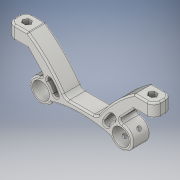
# Autodesk Inventor part: Carbon fibre tube front bracket 3.0
Saved by Autodesk Inventor 2016 (Build 200138000, 138)
## iProperties
Created: 2016-01-16
Part Number: Carbon fibre tube front bracket 3.0
Material: Generic
Document SubType Name: Modeling
Designer: Josiah Stark
Density: 1 g/cm^3
Appearance: Default
Author: Josiah Stark
Autodesk Inventor part; units mm, degrees
ref_plane "YZ Plane" through (0, 0, 0) normal (1, 0, 0) x (0, 1, 0)
sketch "Sketch1" plane through (0, 0, 0) normal (0, 0, 1) x (1, 0, 0)
  line L0 (28.2839, 10) -> (-28.2839, 10)
  circle A0 centre (-38.25, 5) radius 8.15
  circle A1 centre (38.25, 5) radius 8.15
  arc A2 (-28.2839, 10) -> (-28.2839, 0) centre (-38.25, 5) ccw
  arc A3 (28.2839, 0) -> (28.2839, 10) centre (38.25, 5) ccw
  arc A4 (28.2839, 0) -> (-28.2839, 0) centre (0, -97.5837) ccw
  point P0 (0, 0)
  dimension "d4" = 16.3
  dimension "d5" = 3
  dimension "d7" = 101.6
  constraints: 6 point on circle, 5 centre point, 2 end point
  measures "d4" diameter of A1
  measures "d5" radial gap between concentric circles of A0 A2
  measures "d7" radius of A4
extrude "Extrusion1" add sketch "Sketch1" along normal blind 17.5
sketch "Sketch2" plane through (0, 0, 17.5) normal (0, 0, 1) x (1, 0, 0)
  line L0 (70, 33.9014) -> (70, 46.9014)
  line L1 (-70, 46.9014) -> (-70, 33.9014)
  line L2 (28.2839, 10) -> (-28.2839, 10) projected
  line L3 (-70, 46.9014) -> (-50.95, 46.9014)
  line L4 (-50.95, 33.9014) -> (-70, 33.9014)
  line L5 (-70, 33.9014) -> (-70, 46.9014)
  line L6 (70, 46.9014) -> (50.95, 46.9014)
  line L7 (50.95, 33.9014) -> (70, 33.9014)
  line L8 (70, 33.9014) -> (70, 46.9014)
  arc A0 (-28.2839, 10) -> (-28.2839, 0) centre (-38.25, 5) ccw projected
  line L9 (-50.95, 33.9014) -> (-28.2839, 10)
  line L10 (-28.2839, 10) -> (-15.2791, 10)
  arc A1 (-15.2791, 10) -> (-50.95, 46.9014) centre (-122.5432, -57.9958) ccw
  line L11 (50.95, 33.9014) -> (28.2839, 10)
  line L12 (28.2839, 10) -> (15.2791, 10)
  arc A2 (50.95, 46.9014) -> (15.2791, 10) centre (122.5432, -57.9958) ccw
  line L13 (70, 46.9014) -> (50.95, 46.9014)
  line L14 (-50.95, 46.9014) -> (-70, 46.9014)
  line L15 (-70, 33.9014) -> (-50.95, 33.9014)
  line L16 (50.95, 33.9014) -> (70, 33.9014)
  point P0 (0, 0)
  constraints: 32 end point, 7 parallel, 6 horizontal, 4 point on circle, 2 centre point, 2 perpendicular
extrude "Extrusion2" add sketch "Sketch2" against normal blind 17.5
fillet "Fillet1" radius 6.35 2 edges at (-15.2791, 10, 8.75) (15.2791, 10, 8.75)
fillet "Fillet2" radius 2.54 2 edges at (-32.7286, 14.687, 8.75) (32.7286, 14.687, 8.75)
fillet "Fillet3" radius 6.35 4 edges at (-70, 40.4014, 17.5) (-70, 40.4014, 0) (70, 40.4014, 17.5) (70, 40.4014, 0)
fillet "Fillet4" radius 1.524 46 edges at (-68.1401, 46.9014, 15.6401) (-70, 46.9014, 8.75) (-68.1401, 46.9014, 1.8599) (-57.3, 46.9014, 0) (-57.3, 46.9014, 17.5) (68.1401, 46.9014, 15.6401) (70, 46.9014, 8.75) (68.1401, 46.9014, 1.8599) (57.3, 46.9014, 0) (57.3, 46.9014, 17.5) (14.828, 10.7463, 17.5) (0, 10, 17.5) (-14.828, 10.7463, 17.5) (-32.4049, 31.4698, 17.5) (32.4049, 31.4698, 17.5) (14.828, 10.7463, 0) (0, 10, 0) (-14.828, 10.7463, 0) (-32.4049, 31.4698, 0) (32.4049, 31.4698, 0) (-37.5367, 17.7289, 17.5) (-47.3614, -1.4268, 17.5) (-44.5172, 27.118, 17.5) (-37.5367, 17.7289, 0) (-47.3614, -1.4268, 0) (-44.5172, 27.118, 0) (-68.1401, 33.9014, 15.6401) (-70, 33.9014, 8.75) (-68.1401, 33.9014, 1.8599) (-57.3, 33.9014, 0) (-57.3, 33.9014, 17.5) (37.5367, 17.7289, 17.5) (47.3614, -1.4268, 17.5) (44.5172, 27.118, 17.5) (37.5367, 17.7289, 0) (47.3614, -1.4268, 0) (44.5172, 27.118, 0) (68.1401, 33.9014, 15.6401) (70, 33.9014, 8.75) (68.1401, 33.9014, 1.8599) (57.3, 33.9014, 0) (57.3, 33.9014, 17.5) (0, 4.0163, 17.5) (0, 4.0163, 0) (-50.95, 46.9014, 8.75) (50.95, 46.9014, 8.75)
sketch "Sketch3" plane through (0, 0, 17.5) normal (0, 0, 1) x (1, 0, 0)
  circle A0 centre (-38.25, 5) radius 8.15 projected
  line L0 (-38.25, 0) -> (-38.25, 13.15)
  line L1 (0, 13.15) -> (0, 0)
  arc A1 (-18.3779, 11.9601) -> (-51.4221, 45.3774) centre (-122.5432, -57.9958) ccw projected
  line L2 (0, 0) -> (-19.187, 0)
  line L3 (-19.187, 0) -> (-19.187, 13.15)
  line L4 (-19.187, 13.15) -> (0, 13.15)
  line L5 (0, 13.15) -> (0, 0)
  line L6 (-30.1, 0) -> (-30.1, 5)
  line L7 (0, 13.15) -> (0, 0)
  line L8 (-30.1, 5) -> (-30.1, 0)
  arc A2 (-28.0245, 18.6092) -> (-32.1755, 15.6808) centre (-30.1, 17.145) ccw
  line L9 (-19.187, 0) -> (-19.187, 8.89)
  line L10 (-21.6106, 8.89) -> (-21.7362, 8.89)
  arc A3 (-26.7371, 8.2611) -> (-22.2007, 10.3542) centre (-24.2762, 8.89) ccw
  arc A4 (-26.3517, 7.4258) -> (-32.1755, 15.6808) centre (-49.6039, -2.7965) ccw
  arc A5 (-22.2007, 10.3542) -> (-28.0245, 18.6092) centre (-45.453, 0.132) ccw
  line L11 (-19.187, 13.15) -> (0, 13.15)
  line L12 (-19.187, 13.15) -> (0, 13.15)
  point P0 (-30.1, 13.4749)
  point P1 (-24.2762, 6.35)
  point P2 (-24.2762, 11.43)
  point P3 (-29.8335, 13.15)
  point P4 (-23.6426, 13.15)
  point P5 (-24.2762, 14.1572)
  point P6 (-27.1853, 17.78)
  dimension "d28" = 5.08
  dimension "d29" = 5.08
  dimension "d33" = 25.4
  dimension "d34" = 25.4
  constraints: 26 end point, 22 point on circle, 4 centre point, 4 parallel, 1 horizontal, 1 perpendicular, 1 point on line
  measures "d28" diameter of A2
  measures "d29" diameter of A3
  measures "d33" radius of A4
  measures "d34" radius of A5
extrude "Extrusion3" cut sketch "Sketch3" against normal blind 17.5 contours A5 A3 A4 A2 | A4 A3
ref_plane "Work Plane1" through (0, 10, 15.976) normal (-1, 0, 0) x (0, -1, 0)
mirror "Mirror1" about plane through (0, 10, 15.976) normal (-1, 0, 0) of "Extrusion3"
fillet "Fillet6" radius 1.27 24 edges at (-31.5642, 19.2205, 17.5) (-29.1176, 12.2192, 17.5) (-24.6981, 14.7742, 17.5) (-23.2121, 6.5837, 17.5) (-29.1176, 12.2192, 0) (-23.2121, 6.5837, 0) (-24.6981, 14.7742, 0) (-31.5642, 19.2205, 0) (23.2121, 6.5837, 17.5) (24.6981, 14.7742, 17.5) (29.1176, 12.2192, 17.5) (32.1755, 15.6808, 8.75) (31.5642, 19.2205, 17.5) (31.5642, 19.2205, 0) (24.6981, 14.7742, 0) (23.2121, 6.5837, 0) (29.1176, 12.2192, 0) (26.7371, 8.2611, 8.75) (22.2007, 10.3542, 8.75) (28.0245, 18.6092, 8.75) (-22.2007, 10.3542, 8.75) (-26.7371, 8.2611, 8.75) (-32.1755, 15.6808, 8.75) (-28.0245, 18.6092, 8.75)
ref_plane "Work Plane3" through (-4.3057, 60.5338, 15.976) normal (0.7256095, -0.6881067, 0) x (0, 0, -1)
sketch "Sketch6" plane through (-4.3057, 60.5338, 15.976) normal (0.7256095, -0.6881067, 0) x (0, 0, -1)
  line L0 (14.452, 18.6971) -> (14.452, 0) projected
  line L1 (14.452, 18.6971) -> (0, 18.6971)
  line L2 (0, 18.6971) -> (0, 0)
  line L3 (0, 0) -> (14.452, 0)
  line L4 (14.452, 0) -> (14.452, 18.6971)
  line L5 (14.452, 0) -> (0, 0) projected
  line L6 (15.976, -71.8032) -> (-1.524, -71.8032) projected
  circle A0 centre (7.226, -64.7048) radius 1.905
  line L7 (7.226, 0) -> (7.226, -62.7998)
  line L8 (7.226, -66.6098) -> (7.226, -71.8032)
  line L9 (7.226, -71.8032) -> (7.226, -66.6098)
  line L10 (7.226, -62.7998) -> (7.226, -57.6064)
  point P0 (15.976, -40.9611)
  dimension "d45" = 3.81
  constraints: 16 end point, 2 midpoint, 2 parallel, 2 point on circle, 1 centre point, 1 horizontal, 1 perpendicular, 1 point on line
  measures "d45" diameter of A0
extrude "Extrusion5" cut sketch "Sketch6" along normal blind 25.4 contours A0
mirror "Mirror2" about plane through (0, 10, 15.976) normal (-1, 0, 0) of "Extrusion5"
sketch "Sketch7" plane through (51.4221, 46.9014, 1.524) normal (0, 1, 0) x (1, 0, 0)
  line L0 (0, -15.976) -> (-33.0442, -15.976) projected
  line L1 (10.7257, 1.747) -> (-1.2527, 1.747)
  line L2 (-1.2527, 1.747) -> (-1.2527, -15.976)
  line L3 (18.5779, -4.826) -> (18.5779, -9.626) projected
  line L4 (8.8571, -4.051) -> (10.8383, -4.051)
  line L5 (8.8571, -4.051) -> (6.8759, -4.051)
  line L6 (8.8571, -10.655) -> (6.8759, -10.655)
  line L7 (8.8571, -10.655) -> (10.8383, -10.655)
  line L8 (10.8383, -10.655) -> (12.9372, -7.4908)
  line L9 (10.8383, -4.051) -> (12.9372, -7.4908)
  line L10 (4.6833, -7.353) -> (6.8759, -4.051)
  line L11 (4.6833, -7.353) -> (6.8759, -10.655)
  line L12 (18.9668, -16.453) -> (18.9668, -4.051)
  line L13 (0, -15.976) -> (12.2279, -15.976) projected
  point P0 (-51.4221, 1.524)
  dimension "d58" = 6.604
  dimension "d61" = 8.255
  dimension "d62" = 5.321
  constraints: 22 end point, 5 horizontal, 4 point on line, 1 parallel, 1 perpendicular
  measures "d58" distance of L4.start L6.start
  measures "d61" distance of L8.end L10.start
  measures "d62" distance from line of L13 L6.start
extrude "Extrusion6" cut sketch "Sketch7" against normal blind 15.24
mirror "Mirror3" about plane through (0, 0, 0) normal (1, 0, 0) of "Extrusion6"
body "Solid1"
